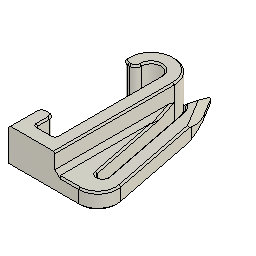
curtainhook30mm v1 (Autodesk Fusion 360 design; units mm, degrees)
Autodesk Fusion 360 part; units mm, degrees
sketch "Sketch2" plane through (0, 0, 0) normal (0, 0, 1) x (1, 0, 0)
  line L0 (0, 0) -> (5, 0)
  line L1 (5, 0) -> (5, -30.1)
  line L2 (5, -30.1) -> (0, -30.1)
  line L3 (0, -30.1) -> (0, 0)
  line L4 (-3.5, -33.6) -> (8.5, -33.6)
  line L5 (8.5, -33.6) -> (8.5, 3.5)
  line L6 (8.5, 3.5) -> (-3.5, 3.5)
  line L7 (-3.5, 3.5) -> (-3.5, -33.6)
  line L8 (-3.5, -25.1) -> (0, -25.1)
  line L9 (-3.5, -4.1) -> (0, -4.1)
  dimension "d12" = 30.1
  dimension "d13" = 5
  dimension "d22" = 3.5
  dimension "d23" = 3.5
  dimension "d24" = 3.5
  dimension "d25" = 3.5
  dimension "d26" = 21
  dimension "d27" = 5
  constraint horizontal L0
  constraint vertical L1
  constraint horizontal L2
  constraint vertical L3
  constraint coincident L0.start L3.end
  constraint horizontal L4
  constraint vertical L5
  constraint horizontal L6
  constraint vertical L7
  constraint coincident L7 L8.start
  constraint perpendicular L7 L8
  constraint coincident L7 L9.start
  constraint coincident L3 L9.end
  constraint perpendicular L3 L9
  measures "d12" distance of L0.start L2.end
  measures "d13" distance of L0.start L0.end
  measures "d22" distance of L3 L7
  measures "d23" distance of L2 L4
  measures "d24" distance of L1 L5
  measures "d25" distance of L0 L6
  measures "d26" distance of L8 L9
  measures "d27" distance of L2 L8.end
extrude "Extrude1" add sketch "Sketch2" along normal blind 9 contours L0 L1 L2 L3 L4 L5 L6 L7 L8 L9
fillet "Fillet1" radius 2.5 2 edges at (5, 0, 4.5) (0, 0, 4.5)
fillet "Fillet1" radius 6 2 edges at (8.5, 3.5, 4.5) (-3.5, 3.5, 4.5)
fillet "Fillet1" radius 1.5 4 edges at (0, -4.1, 4.5) (-3.5, -4.1, 4.5) (0, -25.1, 4.5) (-3.5, -25.1, 4.5)
fillet "Fillet1" radius 0.5 2 edges at (0, -30.1, 4.5) (5, -30.1, 4.5)
sketch "Sketch3" plane through (0, 0, 0) normal (0, 0, -1) x (1, 0, 0)
  arc A0 (-3.5, 26.6) -> (-2, 25.1) centre (-2, 26.6) ccw
  line L0 (-2, 25.1) -> (-1.5, 25.1)
  arc A1 (-1.5, 25.1) -> (0, 26.6) centre (-1.5, 26.6) ccw
  line L1 (0, 26.6) -> (0, 29.6)
  line L2 (0.5, 30.1) -> (4.5, 30.1)
  line L3 (5, 29.6) -> (5, 2.5)
  arc A2 (0, 2.5) -> (5, 2.5) centre (2.5, 2.5) ccw
  line L4 (0, 2.5) -> (0, 2.6)
  arc A3 (0, 2.6) -> (-1.5, 4.1) centre (-1.5, 2.6) ccw
  line L5 (-1.5, 4.1) -> (-2, 4.1)
  arc A4 (-2, 4.1) -> (-3.5, 2.6) centre (-2, 2.6) ccw
  line L6 (-3.5, 2.6) -> (-3.5, 2.5)
  arc A5 (-3.5, 2.5) -> (8.5, 2.5) centre (2.5, 2.5) ccw
  line L7 (8.5, 2.5) -> (8.5, 33.6)
  line L8 (8.5, 33.6) -> (-3.5, 33.6)
  line L9 (-3.5, 33.6) -> (-3.5, 26.6)
  line L10 (8.5, 27.6) -> (16.0491, 27.6) construction
  line L11 (13.5, 27.6) -> (8.5, 2.5)
  line L12 (16.0491, 27.6) -> (10.5511, 0)
  line L13 (0, 0) -> (10.5511, 0) construction
  line L14 (19.6179, 27.6) -> (14.4496, 1.6553)
  line L15 (8.402, 0) -> (9.8492, -5.9212)
  line L16 (8.402, 0) -> (10.8809, 1.6553)
  line L17 (14.4496, 1.6553) -> (9.8492, -5.9212)
  line L18 (14.4496, 1.6553) -> (10.8809, 1.6553) construction
  arc A6 (19.6179, 27.6) -> (14.6952, 33.6) centre (14.6952, 28.5806) ccw
  line L19 (14.6952, 33.6) -> (8.5, 33.6)
  line L20 (8.5, 2.5) -> (8.002, 0)
  line L21 (19.6179, 27.6) -> (16.0491, 27.6) construction
  circle A7 centre (14.7259, 27.3558) radius 1.25
  arc A8 (0.5, 30.1) -> (0, 29.6) centre (0.5, 29.6) ccw
  arc A9 (5, 29.6) -> (4.5, 30.1) centre (4.5, 29.6) ccw
  dimension "d36" = 2.5
  dimension "d37" = 2.5
  dimension "d38" = 5
  dimension "d39" = 3.5
  dimension "d40" = 45
  dimension "d41" = 110
  dimension "d44" = 20
  dimension "d45" = 0.4
  constraint coincident L7 L10.start
  constraint perpendicular L7 L10
  constraint coincident L10 L11.start
  constraint parallel L11 L12
  constraint coincident L13.start origin
  constraint horizontal L13
  constraint coincident L12.end L13.end
  constraint parallel L12 L14
  constraint coincident L12 L16.end
  constraint coincident L13 L15.start
  constraint horizontal L18
  constraint tangent L14 A6
  constraint coincident L7.end L8.start
  constraint perpendicular L7 L19
  constraint tangent A6 L19
  constraint coincident L13 L20.end
  constraint parallel L11 L20
  constraint coincident A5 L7.start
  constraint horizontal L21
  constraint coincident A5.end L7.start
  constraint coincident L11.start A7
  constraint tangent L11 A7
  constraint tangent L12 A7
  measures "d36" distance of L2 L10
  measures "d37" distance of L11 L12
  measures "d38" distance of L10.start L11.start
  measures "d39" distance of L12 L14
  measures "d40" angle of L12 L16
  measures "d41" angle of L15 L16
  measures "d44" angle of L14 L17
  measures "d45" distance of L15.start L20.end
extrude "Extrude2" add sketch "Sketch3" against normal blind 4 contours L7 L11 L12 L14 L15 L16 L17 A6 L19 A7
chamfer "Chamfer1" distance 1 angle 45 1 edges at (8.5, -18.05, 4)
chamfer "Chamfer4" distance 1.6 angle 45 4 edges at (9.1256, 2.9606, 4) (12.1494, 2.133, 4) (12.1494, 2.133, 0) (9.1256, 2.9606, 0)
fillet "Fillet3" radius 0.4 1 edges at (9.8492, 5.9212, 2)
fillet "Fillet3" radius 17 1 edges at (14.4496, -1.6553, 2)
fillet "Fillet3" radius 3 1 edges at (10.8809, -1.6553, 2)
fillet "Fillet3" radius 0.65 1 edges at (8.402, 0, 2)
chamfer "Chamfer5" distance 0.4 angle 45 9 edges at (18.5757, -31.7643, 4) (17.4907, -16.9216, 4) (12.0976, -33.6, 4) (11.5, -17.56, 4) (9.8327, -0.9554, 4) (10.6754, -1.7927, 4) (13.5377, -14.9928, 4) (14.9701, -28.5817, 4) (9, -5.01, 4.5)
chamfer "Chamfer5" distance 0.4 angle 45 24 edges at (17.4907, -16.9216, 0) (5.5976, -33.6, 0) (18.5757, -31.7643, 0) (-3.5, -30.1, 0) (2.5, 3.5, 0) (-3.5, -2.55, 0) (-3.0607, -3.6607, 0) (-1.75, -4.1, 0) (-0.4393, -3.6607, 0) (0, -2.55, 0) (2.5, 0, 0) (5, -16.05, 0) (4.8536, -29.9536, 0) (2.5, -30.1, 0) (0.1464, -29.9536, 0) (0, -28.1, 0) (-0.4393, -25.5393, 0) (-1.75, -25.1, 0) (-3.0607, -25.5393, 0) (11, -15.05, 0) (9.8327, -0.9554, 0) (10.6754, -1.7927, 0) (13.5377, -14.9928, 0) (14.9701, -28.5817, 0)
chamfer "Chamfer5" distance 0.4 angle 45 17 edges at (2.5, 0, 9) (0, -2.55, 9) (-0.4393, -3.6607, 9) (-1.75, -4.1, 9) (-3.0607, -3.6607, 9) (-3.5, -2.55, 9) (2.5, 3.5, 9) (8.5, -18.05, 9) (-3.5, -30.1, 9) (-3.0607, -25.5393, 9) (-1.75, -25.1, 9) (-0.4393, -25.5393, 9) (0, -28.1, 9) (0.1464, -29.9536, 9) (2.5, -30.1, 9) (4.8536, -29.9536, 9) (5, -16.05, 9)
equation "slot_height = 30.1 mm"
equation "slot_width = 5 mm"
equation "hook_offset = 2.5 mm"
equation "hook_slot = 2.5 mm"
equation "track_gap = 21 mm"
equation "body_width = 3.5 mm"
equation "d22 = body_width"
equation "d23 = body_width"
equation "d24 = body_width"
equation "d25 = body_width"
equation "d26 = track_gap"
equation "d36 = hook_offset"
equation "d37 = hook_slot"
equation "d39 = body_width"
equation "d40 = 45 °"
equation "d41 = 110 °"
equation "d44 = 20 °"
named bodies: "hook"
